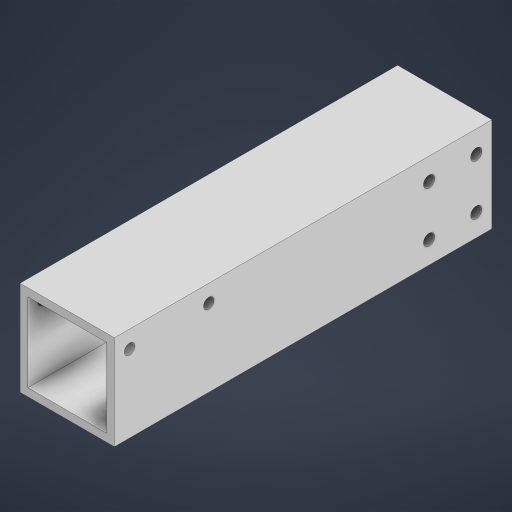
# Autodesk Inventor part: CS_Climb_Outer_Tube
Saved by Autodesk Inventor 2023 (Build 270158000, 158)
## iProperties
Created: 2024-02-19
Part Number: CS_Climb_Outer_Tube
Material: Generic
Document SubType Name: Modeling
Designer: kelle
Density: 1 g/cm^3
Appearance: Default
Author: kelle
Autodesk Inventor part; units mm, degrees
ref_plane "YZ Plane" through (0, 0, 0) normal (1, 0, 0) x (0, 1, 0)
ref_plane "XZ Plane" through (0, 0, 0) normal (0, 1, 0) x (-1, 0, 0)
ref_plane "XY Plane" through (0, 0, 0) normal (0, 0, 1) x (1, 0, 0)
sketch "Sketch1" plane through (0, 0, 0) normal (0, 0, 1) x (1, 0, 0)
  line L0 (19.05, -19.05) -> (-19.05, -19.05)
  line L1 (-19.05, -19.05) -> (-19.05, 19.05)
  line L2 (-19.05, 19.05) -> (19.05, 19.05)
  line L3 (19.05, 19.05) -> (19.05, -19.05)
  line L4 (19.05, -19.05) -> (-19.05, 19.05) construction
  line L5 (-19.05, -19.05) -> (19.05, 19.05) construction
  line L6 (15.875, 15.875) -> (-15.875, 15.875)
  line L7 (-15.875, 15.875) -> (-15.875, -15.875)
  line L8 (-15.875, -15.875) -> (15.875, -15.875)
  line L9 (15.875, -15.875) -> (15.875, 15.875)
  point P0 (0, 0)
  dimension "d0" = 38.1
  dimension "d1" = 38.1
  dimension "d2" = 3.175
  constraints: 20 end point, 4 parallel, 2 midpoint, 2 perpendicular, 1 horizontal, 3 other
  measures "d0" distance of L1.end L2.end
  measures "d1" distance of L0.end L1.end
  measures "d2" distance between parallel lines of L2 L6
extrude "Extrusion1" add sketch "Sketch1" along normal blind 152.4
sketch "Sketch2" plane through (19.05, -19.05, 0) normal (1, 0, 0) x (0, 0, -1)
  line L0 (0, 0) -> (0, 38.1) projected
  line L1 (0, 38.1) -> (-152.4, 38.1) projected
  line L2 (-152.4, 0) -> (-152.4, 38.1) projected
  line L3 (0, 0) -> (-152.4, 0) projected
  line L4 (-76.2, 38.1) -> (-76.2, 0) construction
  line L5 (-152.4, 19.05) -> (0, 19.05) construction
  circle A0 centre (-114.3, 31.115) radius 2.0955
  circle A1 centre (-146.304, 31.115) radius 2.0955
  dimension "d5" = 4.191
  dimension "d7" = 114.3
  dimension "d8" = 4.191
  dimension "d9" = 6.985
  dimension "d10" = 6.985
  dimension "d11" = 32.004
  constraints: 4 end point, 3 midpoint, 2 centre point, 1 perpendicular
  measures "d5" diameter of A0
  measures "d7" distance from line of L0 A0.centre
  measures "d8" diameter of A1
  measures "d9" distance from line of L1 A0.centre
  measures "d10" distance from line of L1 A1.centre
  measures "d11" distance of A0.centre A1.centre
extrude "Extrusion2" cut sketch "Sketch2" against normal through all contours A0 | A1
sketch "Sketch3" plane through (19.05, -19.05, 0) normal (1, 0, 0) x (0, 0, -1)
  line L0 (0, 38.1) -> (-152.4, 38.1) construction
  line L1 (-76.2, 38.1) -> (-76.2, 0) construction
  line L2 (0, 0) -> (-152.4, 0) construction
  line L3 (0, 19.05) -> (-152.4, 19.05) construction
  line L4 (-152.4, 38.1) -> (-152.4, 0) construction
  circle A0 centre (-6.35, 29.21) radius 2.25
  line L5 (0, 0) -> (0, 38.1) projected
  circle A1 centre (-6.35, 8.89) radius 2.25
  circle A2 centre (-25.4, 29.21) radius 2.25
  circle A3 centre (-25.4, 8.89) radius 2.25
  dimension "d14" = 4.5
  dimension "d15" = 6.35
  dimension "d16" = 4.5
  dimension "d17" = 6.35
  dimension "d18" = 8.89
  dimension "d19" = 8.89
  dimension "d20" = 4.5
  dimension "d21" = 19.05
  dimension "d22" = 4.5
  constraints: 4 centre point, 4 end point, 3 midpoint
  measures "d14" diameter of A0
  measures "d15" distance from line of L5 A0.centre
  measures "d16" diameter of A1
  measures "d17" distance from line of L5 A1.centre
  measures "d18" distance from line of L2 A1.centre
  measures "d19" distance from line of L0 A0.centre
  measures "d20" diameter of A2
  measures "d21" distance of A0.centre A2.centre
  measures "d22" diameter of A3
extrude "Extrusion3" cut sketch "Sketch3" against normal through all
body "Solid1"
